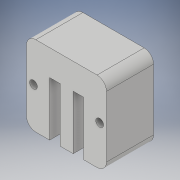
# Autodesk Inventor part: FingerProximalPhanalaxJoint
Saved by Autodesk Inventor 2018 (Build 220112000, 112)
## iProperties
Created: 2018-01-12
Part Number: FingerProximalPhanalaxJoint
Material: Generic
Document SubType Name: Modeling
Designer: iancostello
Density: 1 g/cm^3
Appearance: Default
Author: iancostello
Autodesk Inventor part; units mm, degrees
ref_plane "YZ Plane" through (0, 0, 0) normal (1, 0, 0) x (0, 1, 0)
ref_plane "XZ Plane" through (0, 0, 0) normal (0, 1, 0) x (-1, 0, 0)
ref_plane "XY Plane" through (0, 0, 0) normal (0, 0, 1) x (1, 0, 0)
sketch "Sketch2" plane through (0, 0, 0) normal (0, 1, 0) x (-1, 0, 0)
  line L0 (8.4618, 0) -> (-8.5382, 0)
  line L1 (-8.5382, 0) -> (-8.5382, -10)
  line L2 (-8.5382, -10) -> (8.4618, -10)
  line L3 (8.4618, -10) -> (8.4618, 0)
  line L4 (-0.0382, 13.1242) -> (-0.0382, -17.558) construction
  point P0 (0, 0)
  dimension "d3" = 17
  dimension "d4" = 10
  constraints: 10 end point, 1 vertical, 1 other
  measures "d3" distance of L0.start L0.end
  measures "d4" distance of L1.end L0.end
extrude "Extrusion1" add sketch "Sketch2" along normal blind 8.5 and the other way blind 8.5
sketch "Sketch3" plane through (0, 0, 0) normal (0, 1, 0) x (-1, 0, 0)
  line L0 (-8.5382, -10) -> (8.4618, -10) projected
  circle A0 centre (-0.0382, -10) radius 5.5
  line L1 (5.4618, -10) -> (-0.0382, -10)
  line L2 (-0.0382, -4.5) -> (-0.0382, -10)
  point P0 (0, 0)
  dimension "d9" = 11
  constraints: 4 end point, 2 point on circle, 1 centre point, 1 collinear, 1 midpoint, 1 perpendicular, 1 point on line
  measures "d9" diameter of A0
revolve "Revolution1" cut sketch "Sketch3" angle 360 about axis through (0.0382, 0, -4.5) along (0, 0, -1) picked at (3.0469, -8.0615) contours L2 A0 L0
sketch "Sketch4" plane through (-8.4618, 8.5, 0) normal (0, 0, 1) x (1, 0, 0)
  line L0 (8.5303, -2) -> (8.5303, -5.5) construction
  line L1 (10, -16.5) -> (10, -13) construction
  line L2 (8.5303, -5.5) -> (9.9303, -5.5) construction
  line L3 (9.9303, -5.5) -> (12.1303, -5.5)
  line L4 (12.1303, -5.5) -> (12.1303, -18.7305)
  line L5 (12.1303, -18.7305) -> (9.9303, -18.7305)
  line L6 (9.9303, -18.7305) -> (9.9303, -5.5)
  line L7 (7.1303, -5.5) -> (4.9303, -5.5)
  line L8 (4.9303, -5.5) -> (4.9303, -18.7305)
  line L9 (4.9303, -18.7305) -> (7.1303, -18.7305)
  line L10 (7.1303, -18.7305) -> (7.1303, -5.5)
  line L11 (0, 0) -> (17, 0) projected
  line L12 (8.5, 0) -> (8.5, -17) construction
  line L13 (0, -17) -> (17, -17) projected
  line L14 (9.9303, 0) -> (9.9303, -5.5) construction
  point P0 (8.4618, -8.5)
  dimension "d11" = 3.5
  dimension "d12" = 3.5
  dimension "d20" = 1.4
  dimension "d21" = 2.2
  dimension "d23" = 5.5
  constraints: 26 end point, 4 symmetric about line, 3 vertical, 2 horizontal, 2 midpoint, 2 parallel, 1 coincident, 1 perpendicular, 1 point on line
  measures "d11" distance of L0.start L0.end
  measures "d12" distance of L1.start L1.end
  measures "d20" distance of L2.start L2.end
  measures "d21" distance of L2.end L3.end
  measures "d23" distance of L14.start L14.end
extrude "Extrusion2" cut sketch "Sketch4" against normal blind 10
fillet "Fillet1" radius 2 4 edges at (8.5382, 8.5, -5) (8.5382, -8.5, -5) (-8.4618, -8.5, -5) (-8.4618, 8.5, -5)
sketch "Sketch6" plane through (-1.3315, -8.5, 0) normal (0, 0, 1) x (1, 0, 0)
  arc A0 (5, 4.3683) -> (-2.2, 4.3158) centre (1.3697, 8.5) ccw projected
  line L0 (-4.1303, 8.5) -> (-5.6303, 8.5) construction
  circle A1 centre (-5.6303, 8.5) radius 0.8255
  line L1 (1.4, 0.7279) -> (1.4, 15.8188) construction
  circle A2 centre (8.4303, 8.5) radius 0.8255
  point P0 (1.3315, 8.5)
  dimension "d24" = 1.5
  dimension "d25" = 1.651
  constraints: 4 end point, 2 centre point, 1 coincident, 1 horizontal, 1 point on circle, 1 symmetric about line, 1 vertical, 1 other
  measures "d24" distance of L0.start L0.end
  measures "d25" diameter of A1
extrude "Extrusion4" cut sketch "Sketch6" against normal blind 10
body "Solid1"
